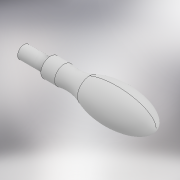
# Autodesk Inventor part: 特征2
Saved by Autodesk Inventor 2020 (Build 240168000, 168)
## iProperties
Created: 2021-03-24
Part Number: 特征2
Material: 常规
Document SubType Name: Sheet Metal
Designer: Luorily
Density: 1 g/cm^3
Sheet Metal Rule: 默认
Appearance: 默认
Author: Luorily
Autodesk Inventor part; units mm, degrees
ref_plane "YZ Plane" through (0, 0, 0) normal (1, 0, 0) x (0, 1, 0)
ref_plane "XZ Plane" through (0, 0, 0) normal (0, 1, 0) x (-1, 0, 0)
ref_plane "XY Plane" through (0, 0, 0) normal (0, 0, 1) x (1, 0, 0)
sketch "草图1" plane through (0, 0, 0) normal (0, 0, 1) x (1, 0, 0)
  line L0 (0, 6) -> (0, 9)
  line L1 (0, 9) -> (13, 9)
  line L2 (0, 0) -> (63, 0)
  arc A0 (13, 9) -> (37.0425, 11.4019) centre (21.1786, 48.6656) ccw
  line L3 (0, 0) -> (100, 0)
  ellipse E0 centre (63, 0) end of major axis (100, 0) minor radius 16 (100, 0) -> (37.0425, 11.4019) ccw
  line L4 (0, 6) -> (-25, 6)
  line L5 (-25, 6) -> (-25, 0)
  line L6 (-25, 0) -> (0, 0)
  dimension "d6" = 16
  dimension "d1" = 13
  dimension "d3" = 81
  dimension "d8" = 25
  constraints: 14 end point, 3 horizontal, 3 perpendicular, 2 point on circle, 1 centre point, 1 coincident, 1 vertical, 5 other
  measures "d1" distance of L0.end L1.end
  measures "d3" diameter of A0
  measures "d8" distance of L0.start L4.end
revolve "旋转1" add sketch "草图1" angle 360 about axis through (0, 0, 0) along (1, 0, 0)
sketch "草图2" plane through (-25, 0, 0) normal (-1, 0, 0) x (0, 0, 1)
  point P0 (0, 0)
  point P1 (0, 0)
  constraints: 1 coincident
hole "孔1" at (-25, 0, 0) direction (1, 0, 0) diameter 9 depth 6 tip angle 118
equation "\"折弯半径\" = 厚度"
equation "\"折弯释压宽度\" = 厚度"
equation "\"折弯释压深度\" = 0.5 * 厚度"
equation "\"拐角释压尺寸\" = 4 * 厚度"
equation "\"最小余量\" = 2 * 厚度"
equation "\"过渡半径\" = 折弯半径"
equation "\"Jacobi半径尺寸\" = 厚度"
equation "\"间隙大小\" = 厚度"
equation "\"厚度\" = 0.5"
